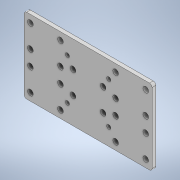
# Autodesk Inventor part: De truc Z
Saved by Autodesk Inventor 2020 (Build 240168000, 168)
## iProperties
Created: 2021-05-25
Part Number: De truc Z
Material: Generic
Document SubType Name: Modeling
Designer: admin
Density: 1 g/cm^3
Appearance: Default
Author: admin
Autodesk Inventor part; units mm, degrees
ref_plane "YZ Plane" through (0, 0, 0) normal (1, 0, 0) x (0, 1, 0)
ref_plane "XZ Plane" through (0, 0, 0) normal (0, 1, 0) x (-1, 0, 0)
ref_plane "XY Plane" through (0, 0, 0) normal (0, 0, 1) x (1, 0, 0)
sketch "Sketch1" plane through (0, 0, 0) normal (0, 0, 1) x (1, 0, 0)
  line L0 (-51, -30) -> (51, -30)
  line L1 (51, -30) -> (51, 30)
  line L2 (51, 30) -> (-51, 30)
  line L3 (-51, 30) -> (-51, -30)
  line L4 (-51, -30) -> (51, 30) construction
  line L5 (51, -30) -> (-51, 30) construction
  point P0 (0, 0)
  dimension "d0" = 102
  dimension "d3" = 60
  constraints: 12 end point, 2 midpoint, 2 parallel, 1 horizontal, 1 perpendicular
  measures "d0" distance of L2.end L1.end
  measures "d3" distance between parallel lines of L0 L2
extrude "Extrusion1" add sketch "Sketch1" along normal blind 3
sketch "Sketch2" plane through (0, 0, 3) normal (0, 0, 1) x (1, 0, 0)
  line L0 (22, -24) -> (46, -24)
  line L1 (46, -24) -> (46, -6)
  line L2 (46, -6) -> (22, -6)
  line L3 (22, -6) -> (22, -24)
  line L4 (22, -24) -> (46, -6) construction
  line L5 (46, -24) -> (22, -6) construction
  line L6 (-51, -30) -> (51, -30) projected
  line L7 (51, -30) -> (51, 30) projected
  circle A0 centre (46, -6) radius 2.25
  circle A1 centre (46, -24) radius 2.25
  circle A2 centre (22, -24) radius 2.25
  circle A3 centre (22, -6) radius 2.25
  point P0 (0, 0)
  point P1 (34, -15)
  dimension "d4" = 24
  dimension "d5" = 18
  dimension "d6" = 15
  dimension "d7" = 5
  dimension "d8" = 4.5
  dimension "d9" = 4.5
  dimension "d10" = 4.5
  dimension "d11" = 4.5
  constraints: 12 end point, 4 centre point, 4 coincident, 2 midpoint, 2 parallel, 1 horizontal, 1 perpendicular
  measures "d4" distance of L2.end L1.end
  measures "d5" distance of L1.end L0.end
  measures "d6" distance from line of L6 point (34, -15)
  measures "d7" distance between parallel lines of L7 L1
  measures "d8" diameter of A0
  measures "d9" diameter of A1
  measures "d10" diameter of A2
  measures "d11" diameter of A3
extrude "Extrusion2" cut sketch "Sketch2" against normal blind 3 contours L3 A2 L0 | L0 A2 L3 | A1 L1 L0 | L0 L1 A1 | A3 L2 L3 | L3 L2 A3 | A0 L2 L1 | L1 L2 A0
pattern_linear "Rectangular Pattern1" count 2 spacing 30 along (0, 1, 0) of "Extrusion2"
sketch "Sketch3" plane through (0, 0, 3) normal (0, 0, 1) x (1, 0, 0)
  line L0 (-12, -9) -> (12, -9)
  line L1 (12, -9) -> (12, 9)
  line L2 (12, 9) -> (-12, 9)
  line L3 (-12, 9) -> (-12, -9)
  line L4 (-12, -9) -> (12, 9) construction
  line L5 (12, -9) -> (-12, 9) construction
  circle A0 centre (-12, 9) radius 2.25
  circle A1 centre (12, 9) radius 2.25
  circle A2 centre (12, -9) radius 2.25
  circle A3 centre (-12, -9) radius 2.25
  point P0 (0, 0)
  dimension "d20" = 24
  dimension "d21" = 18
  dimension "d22" = 4.5
  dimension "d23" = 4.5
  dimension "d24" = 4.5
  dimension "d25" = 4.5
  constraints: 12 end point, 4 centre point, 4 coincident, 2 midpoint, 2 parallel, 1 horizontal, 1 perpendicular
  measures "d20" distance of L2.end L1.end
  measures "d21" distance of L1.end L0.end
  measures "d22" diameter of A0
  measures "d23" diameter of A1
  measures "d24" diameter of A2
  measures "d25" diameter of A3
extrude "Extrusion3" cut sketch "Sketch3" against normal blind 3 contours L3 A3 L0 | L0 A3 L3 | A2 L1 L0 | L0 L1 A2 | A0 L2 L3 | L3 L2 A0 | A1 L2 L1 | L1 L2 A1
sketch "Sketch4" plane through (0, 0, 3) normal (0, 0, 1) x (1, 0, 0)
  line L0 (-16.5, -16.5) -> (16.5, -16.5)
  line L1 (16.5, -16.5) -> (16.5, 16.5)
  line L2 (16.5, 16.5) -> (-16.5, 16.5)
  line L3 (-16.5, 16.5) -> (-16.5, -16.5)
  line L4 (-16.5, -16.5) -> (16.5, 16.5) construction
  line L5 (16.5, -16.5) -> (-16.5, 16.5) construction
  circle A0 centre (16.5, 16.5) radius 1.65
  circle A1 centre (-16.5, 16.5) radius 1.65
  circle A2 centre (-16.5, -16.5) radius 1.65
  circle A3 centre (16.5, -16.5) radius 1.65
  point P0 (0, 0)
  dimension "d28" = 33
  dimension "d29" = 33
  dimension "d30" = 3.3
  dimension "d31" = 3.3
  dimension "d32" = 3.3
  dimension "d33" = 3.3
  constraints: 12 end point, 4 centre point, 4 coincident, 2 midpoint, 2 parallel, 1 horizontal, 1 perpendicular
  measures "d28" distance of L2.end L1.end
  measures "d29" distance of L1.end L0.end
  measures "d30" diameter of A0
  measures "d31" diameter of A1
  measures "d32" diameter of A2
  measures "d33" diameter of A3
extrude "Extrusion4" cut sketch "Sketch4" against normal blind 3 contours L3 A2 L0 | L0 A2 L3 | A3 L1 L0 | L0 L1 A3 | A1 L2 L3 | L3 L2 A1 | A0 L2 L1 | L1 L2 A0
mirror "Mirror1" about plane through (0, 0, 0) normal (1, 0, 0) of "Extrusion2", "Rectangular Pattern1"
fillet "Fillet1" radius 2 4 edges at (51, 30, 1.5) (51, -30, 1.5) (-51, -30, 1.5) (-51, 30, 1.5)
body "Solid1"
